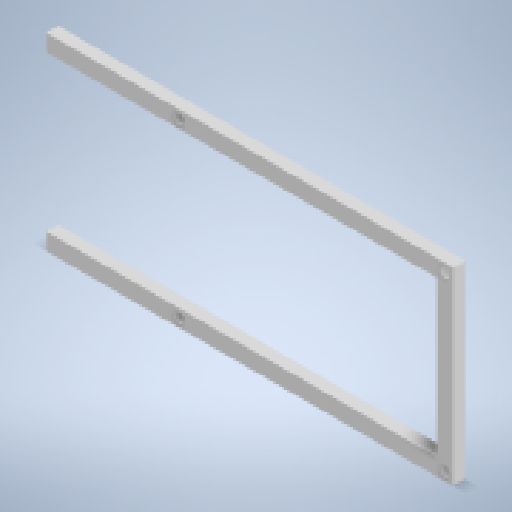
# Autodesk Inventor part: ExtensionMarco
Saved by Autodesk Inventor 2024 (Build 280153000, 153)
## iProperties
Created: 2024-01-06
Part Number: ExtensionMarco
Material: Genérico
Document SubType Name: Modeling
Designer: sergi
Density: 1 g/cm^3
Appearance: Valor por defecto
Author: sergi
Autodesk Inventor part; units mm, degrees
ref_plane "YZ Plane" through (0, 0, 0) normal (1, 0, 0) x (0, 1, 0)
ref_plane "XZ Plane" through (0, 0, 0) normal (0, 1, 0) x (-1, 0, 0)
ref_plane "XY Plane" through (0, 0, 0) normal (0, 0, 1) x (1, 0, 0)
sketch "Boceto1" plane through (0, 0, 0) normal (0, 0, 1) x (1, 0, 0)
  line L0 (0, -32.35) -> (0, -39.35) projected
  line L1 (0, -39.35) -> (169, -39.35) projected
  arc A0 (169, -39.35) -> (169.5, -38.85) centre (169, -38.85) ccw projected
  line L2 (169.5, -38.85) -> (169.5, 38.85) projected
  arc A1 (169.5, 38.85) -> (169, 39.35) centre (169, 38.85) ccw projected
  line L3 (169, 39.35) -> (0, 39.35) projected
  line L4 (0, 39.35) -> (0, 32.35) projected
  line L5 (0, 32.35) -> (162.5, 32.35) projected
  line L6 (162.5, 32.35) -> (162.5, -32.35) projected
  line L7 (162.5, -32.35) -> (0, -32.35) projected
  circle A2 centre (166, 35.85) radius 2.15 projected
  circle A3 centre (166, -35.85) radius 2.15 projected
  circle A4 centre (55.3333, 35.85) radius 2.15 projected
  circle A5 centre (55.3333, -35.85) radius 2.15 projected
  point P0 (0, 0)
extrude "Extrusión1" add sketch "Boceto1" along normal blind 5
